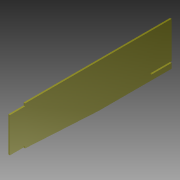
# Autodesk Inventor part: window
Saved by Autodesk Inventor 2014 SP2 (Build 180246200, 246)
## iProperties
Created: 2016-05-05
Part Number: window
Material: Generic
Document SubType Name: Modeling
Designer: cruiser
Density: 1 g/cm^3
Appearance: Clear - Yellow
Author: cruiser
Autodesk Inventor part; units mm, degrees
ref_plane "YZ Plane" through (0, 0, 0) normal (1, 0, 0) x (0, 1, 0)
ref_plane "XZ Plane" through (0, 0, 0) normal (0, 1, 0) x (-1, 0, 0)
ref_plane "XY Plane" through (0, 0, 0) normal (0, 0, 1) x (1, 0, 0)
sketch "Sketch2" plane through (0, 0, 0) normal (1, 0, 0) x (0, 1, 0)
  line L0 (144.9563, -38.5312) -> (-144.9563, -38.5313)
  line L1 (-144.9563, -38.5313) -> (-144.9563, 38.5312)
  line L2 (-144.9563, 38.5312) -> (144.9563, 38.5313)
  line L3 (144.9563, 38.5313) -> (144.9563, -38.5312)
  line L4 (144.9563, -38.5312) -> (-144.9563, 38.5312) construction
  line L5 (-144.9563, -38.5313) -> (144.9563, 38.5313) construction
  line L6 (-144.9563, 33.5312) -> (-174.9563, 33.5312)
  line L7 (-174.9563, 33.5312) -> (-174.9563, -35.3563)
  line L8 (-174.9563, -35.3563) -> (-144.9563, -35.3563)
  line L9 (-144.9563, -35.3563) -> (-144.9563, 33.5312)
  line L10 (144.9563, -38.5312) -> (0, -38.5312)
  line L11 (0, -38.5312) -> (0, -46.9438)
  line L12 (0, -46.9438) -> (144.9563, -46.9437)
  line L13 (144.9563, -46.9437) -> (144.9563, -38.5312)
  line L14 (0, 0) -> (0, -38.5312)
  line L15 (0, -46.9438) -> (-144.9563, -38.5313)
  dimension "d0" = 289.9125
  dimension "d1" = 77.0625
  dimension "d6" = 3.175
  dimension "d7" = 5
  dimension "d8" = 30
  dimension "d9" = 8.4125
  dimension "d17" = 0
  constraints: 32 end point, 6 parallel, 3 horizontal, 3 midpoint, 3 perpendicular, 1 collinear
  measures "d0" distance of L1.end L2.end
  measures "d1" distance of L0.end L1.end
  measures "d6" distance between parallel lines of L0 L8
  measures "d7" distance between parallel lines of L2 L6
  measures "d8" distance between parallel lines of L1 L7
  measures "d9" distance between parallel lines of L0 L12
  measures "d17" distance between parallel lines of L14 L11
extrude "Extrusion1" add sketch "Sketch2" along normal blind 3.15
sketch "Sketch3" plane through (3.15, 0, 0) normal (1, 0, 0) x (0, 0, -1)
  line L0 (46.9438, 0) -> (46.9437, 144.9563) projected
  line L1 (46.9437, 144.9563) -> (-38.5313, 144.9563) projected
  line L2 (33.7937, 144.9563) -> (36.9437, 144.9563)
  line L3 (36.9437, 144.9563) -> (36.9437, 104.9563)
  line L4 (36.9437, 104.9563) -> (33.7937, 104.9563)
  line L5 (33.7937, 104.9563) -> (33.7937, 144.9563)
  point P0 (0, 0)
  dimension "d11" = 40
  dimension "d12" = 3.15
  dimension "d13" = 10
  constraints: 8 end point, 2 parallel, 1 horizontal, 1 perpendicular, 1 point on line
  measures "d11" distance of L4.end L2.start
  measures "d12" distance between parallel lines of L3 L5
  measures "d13" distance between parallel lines of L0 L3
extrude "Extrusion2" cut sketch "Sketch3" against normal blind 10
equation "\"d0\" = window_z"
equation "\"d1\" = window_y"
equation "\"d6\" = 2 * sm_thickness"
equation "\"d7\" = acrylic_into_frame"
equation "\"d8\" = window_overlap"
equation "\"d9\" = protection_slot_width - sm_thickness"
equation "\"d2\" = clear_acrylic"
equation "\"d11\" = 0.5 * protection_slot_length"
equation "\"d12\" = clear_acrylic"
equation "\"d13\" = protection_slot_width"
equation "\"sm_thickness\" = 1.5875"
equation "\"very_thick_acrylic\" = 9.45"
equation "\"thick_acrylic\" = 5.88"
equation "\"thin_acrylic\" = 3.15"
equation "\"clear_acrylic\" = 3.15"
equation "\"wood_thickness\" = 6.72"
equation "\"m3_diameter\" = 3.15"
equation "\"m4_diameter\" = 4.2"
equation "\"m5_diameter\" = 5.25"
equation "\"brass_insert_drill\" = 4"
equation "\"m5_brass_insert_drill\" = 6.7"
equation "\"m3_main_length\" = 14"
equation "\"m3_main_nut_width\" = 5.7"
equation "\"m3_main_nut_thickness\" = 2.5"
equation "\"m3_main_extra\" = 1"
equation "\"stepper_screw_space\" = 35"
equation "\"stepper_shaft_diameter\" = 5"
equation "\"stepper_body_diameter\" = 28"
equation "\"laser_body_diameter\" = 12"
equation "\"carrier_y\" = 221"
equation "\"carrier_z\" = 12"
equation "\"visor_x\" = 227.3"
equation "\"visor_y\" = 90.5"
equation "\"protection_slot\" = 44.2"
equation "\"protection_slot_offset\" = 55.25"
equation "\"window_z\" = 289.9125"
equation "\"bed_z2\" = 74.6"
equation "\"crane_z\" = 45"
equation "\"bed_z\" = 25.4"
equation "\"bed_y\" = 141"
equation "\"reservoir_x\" = 181"
equation "\"crane_z2\" = 12"
equation "\"end_stop_offset_x\" = 47"
equation "\"tray_y\" = 221"
equation "\"door_sensor\" = 35"
equation "\"linear_bearing_spacing\" = 247"
equation "\"bed_x\" = 141"
equation "\"motor_spacing\" = 327"
equation "\"tray_x\" = 221"
equation "\"reservoir_y\" = 181"
equation "\"window_y\" = 77.0625"
equation "\"end_stop_spacing\" = 19"
equation "\"threaded_rod_z\" = 203.2"
equation "\"window_overlap\" = 30"
equation "\"door_z\" = 289.9125"
equation "\"door_x\" = 221"
equation "\"acrylic_into_frame\" = 5"
equation "\"protection_slot_width\" = 10"
equation "\"protection_slot_length\" = 80"
body "Solid1"
